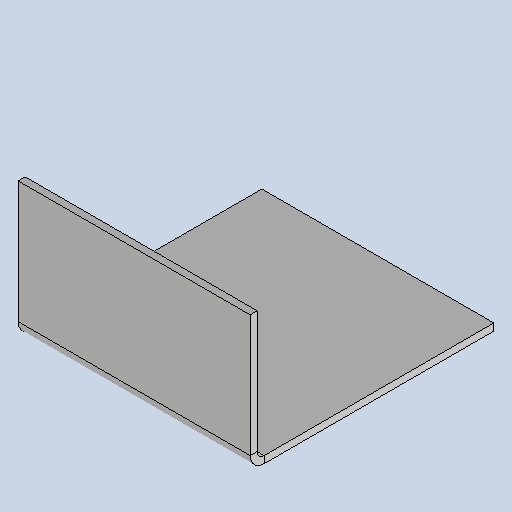
# Autodesk Inventor part: PRS 9672 charging tube 2_D1200 940
Saved by Autodesk Inventor 2026.2 (Build 302298010, 298A)
## iProperties
Created: 2025-02-13
Part Number: PRS 9672 charging tube 2_D1200 940
Material: Steel
Document SubType Name: Sheet Metal
Designer: admin
Mass: 2466.79 g
Surface Area: 934.137 cm^2
Volume: 314.241 cm^3
Density: 7.85 g/cm^3
Flat Pattern Width: 31.3572 cm
Flat Pattern Length: 19.8 cm
Flat Pattern Area: 620.872 cm^2
Sheet Metal Rule: AISI304 4mm Die 32
Sheet Metal Width: 313,572 mm
Sheet Metal Length: 198,000 mm
Sheet Metal Area: 62087,193 mm^2
Appearance: Default
Author: pokla
Autodesk Inventor part; units mm, degrees
ref_plane "YZ Plane" through (0, 0, 0) normal (1, 0, 0) x (0, 1, 0)
ref_plane "XZ Plane" through (0, 0, 0) normal (0, 1, 0) x (-1, 0, 0)
sketch "Sketch2" plane through (0, 0, 0) normal (0, 0, 1) x (1, 0, 0)
  line L0 (0, -104) -> (-198, -104)
  line L1 (-198, -104) -> (-198, 104)
  line L2 (-198, 104) -> (0, 104)
  line L3 (0, 104) -> (0, -104)
  point P0 (0, 99)
  point P1 (0, -99)
  point P2 (0, 0)
  dimension "d29" = 198
  dimension "d30" = 208
  dimension "d31" = 5
  dimension "d32" = 5
  measures "d29" distance of L1.end L2.end
  measures "d30" distance of L0.end L1.end
  measures "d31" distance of L2.end point (0, 99)
  measures "d32" distance of L0.start point (0, -99)
extrude "Plate2" add sketch "Sketch2" along normal blind 6
sketch "Sketch5" plane through (0, -98, 0) normal (0, -1, 0) x (1, 0, 0)
  line L0 (-198, 0) -> (0, 0)
  line L1 (0, 0) -> (0, 116)
  line L2 (0, 116) -> (-198, 116)
  line L3 (-198, 116) -> (-198, 0)
  constraints: 6 end point, 1 horizontal, 1 perpendicular, 1 vertical
edge flange "Flange1" height 116 angle 90 thickness 6 bend radius 6 thickness toward (0, -1, 0) relief round relief width 6 relief depth 3 edges at (-99, -104, 6) wall of the first edge with corners at (-198, -98, 0) (0, -98, 0) (0, -98, 116) (-198, -98, 116)
bend "Bend1"
corner "Corner1"
ref_plane "Work Plane2" through (0, -98, 116) normal (0.5, 0, 0.8660254) x (0, -1, 0)
equation "\"d30\" = ChargingHatch_width"
equation "\"d14\" = Thickness"
equation "\"d34\" = BendReliefWidth"
equation "\"d35\" = BendReliefDepth"
equation "\"d36\" = MinimumRemnant"
equation "\"d37\" = TransitionRadius"
equation "\"d38\" = ChargingHatch_hight - Thickness"
equation "\"d40\" = BendRadius"
equation "\"d41\" = CornerReliefSize"
equation "\"d42\" = GapSize"
equation "\"d43\" = JacobiRadiusSize"
equation "\"d32\" = d31"
equation "\"BendReliefWidth\" = Thickness"
equation "\"BendReliefDepth\" = 0.5 * Thickness"
equation "\"CornerReliefSize\" = 4 * Thickness"
equation "\"MinimumRemnant\" = 2 * Thickness"
equation "\"TransitionRadius\" = BendRadius"
equation "\"JacobiRadiusSize\" = BendRadius"
equation "\"GapSize\" = Thickness"
equation "\"ChargingHatch_width\" = 208"
equation "\"Thickness\" = 6"
equation "\"ChargingHatch_hight\" = 122"
equation "\"BendRadius\" = 6"
body "Solid3"
